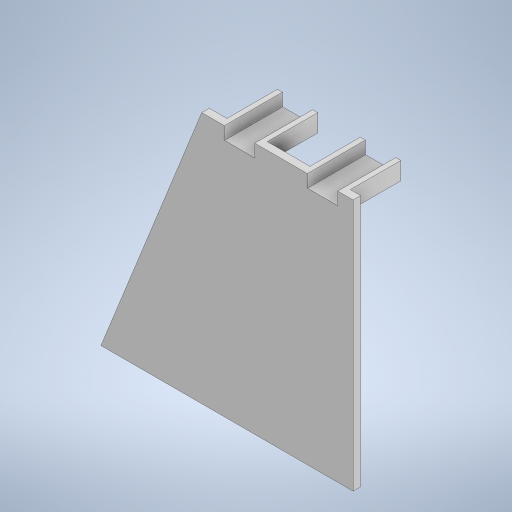
# Autodesk Inventor part: BasePart
Saved by Autodesk Inventor 2024 (Build 280153000, 153)
## iProperties
Created: 2024-03-22
Part Number: BasePart
Material: Generic
Document SubType Name: Modeling
Designer: Wojtek
Density: 1 g/cm^3
Appearance: Default
Author: Wojtek
Autodesk Inventor part; units mm, degrees
ref_plane "YZ Plane" through (0, 0, 0) normal (1, 0, 0) x (0, 1, 0)
ref_plane "XZ Plane" through (0, 0, 0) normal (0, 1, 0) x (-1, 0, 0)
ref_plane "XY Plane" through (0, 0, 0) normal (0, 0, 1) x (1, 0, 0)
sketch "Sketch1" plane through (0, 0, 0) normal (0, 0, 1) x (1, 0, 0)
  line L0 (50, -50) -> (-50, -50)
  line L1 (50, 50) -> (50, -50)
  line L2 (50, 50) -> (-10, 50)
  line L3 (-10, 50) -> (-50, -50)
  line L4 (-10, 50) -> (20, 50)
  line L5 (20, 50) -> (50, 50)
  line L6 (-1, 45) -> (11, 45)
  line L7 (11, 45) -> (11, 55)
  line L8 (11, 55) -> (-1, 55)
  line L9 (-1, 55) -> (-1, 45)
  line L10 (-1, 45) -> (11, 55) construction
  line L11 (11, 45) -> (-1, 55) construction
  line L12 (50, 50) -> (37.9, 50)
  line L13 (31.9, 45) -> (43.9, 45)
  line L14 (43.9, 45) -> (43.9, 55)
  line L15 (43.9, 55) -> (31.9, 55)
  line L16 (31.9, 55) -> (31.9, 45)
  line L17 (31.9, 45) -> (43.9, 55) construction
  line L18 (43.9, 45) -> (31.9, 55) construction
  line L19 (-3, 50) -> (-3, 43)
  line L20 (-3, 43) -> (13, 43)
  line L21 (13, 43) -> (13, 50)
  line L22 (29.9, 50) -> (29.9, 43)
  line L23 (29.9, 43) -> (45.9, 43)
  line L24 (45.9, 43) -> (45.9, 50)
  point P0 (0, 0)
  point P1 (5, 50)
  point P2 (-1, 50)
  point P3 (45.9, 46.5)
  point P4 (31.9, 50)
  point P5 (43.9, 50)
  point P6 (-1, 50)
  point P7 (11, 50)
  dimension "d18" = 60
  dimension "d19" = 111.801
  dimension "d20" = 100
  dimension "d21" = 100
  dimension "d22" = 50
  dimension "d23" = 50
  dimension "d24" = 30
  dimension "d25" = 12
  dimension "d26" = 10
  dimension "d31" = 12.1
  dimension "d32" = 12
  dimension "d33" = 10
  dimension "d36" = 2
  dimension "d37" = 2
  dimension "d38" = 16
  dimension "d39" = 2
  dimension "d40" = 2
  dimension "d41" = 2
  constraints: 50 end point, 8 midpoint, 7 perpendicular, 5 point on line, 4 horizontal, 4 parallel, 1 collinear, 1 vertical
  measures "d18" distance of L1.start L2.end
  measures "d19" angle of L2 L3
  measures "d20" vertical distance of L2.end L0.end
  measures "d21" distance of L0.start L0.end
  measures "d22" horizontal distance of L0.start point (0, 0)
  measures "d23" horizontal distance of point (0, 0) L0.end
  measures "d24" distance of L2.end L4.end
  measures "d25" distance of L8.end L7.end
  measures "d26" distance of L7.end L6.end
  measures "d31" distance of L1.start L12.end
  measures "d32" distance of L15.end L14.end
  measures "d33" distance of L14.end L13.end
  measures "d36" distance between parallel lines of L20 L6
  measures "d37" distance of point (-1, 50) L19.start
  measures "d38" distance from line of L19.start L21
  measures "d39" distance between parallel lines of L16 L22
  measures "d40" distance between parallel lines of L13 L23
  measures "d41" distance from line of point (45.9, 46.5) L14
extrude "Extrusion1" add sketch "Sketch1" along normal blind 3 contours L0 L3 L2 L19 L20 L21 L22 L23 L24 L1 | L24 L23 L22 L2 L16 L13 L14 | L2 L9 L6 L7 L21 L20 L19 | L14 L13 L16 L2 | L2 L7 L6 L9
extrude "Extrusion2" cut sketch "Sketch1" along normal blind 10 contours L9 L8 L7 L2 | L2 L7 L6 L9
extrude "Extrusion3" cut sketch "Sketch1" along normal blind 10 contours L14 L13 L16 L2 | L2 L16 L15 L14
extrude "Extrusion4" add sketch "Sketch1" against normal blind 20 contours L24 L23 L22 L2 L16 L13 L14 | L2 L9 L6 L7 L21 L20 L19
body "Solid1"
